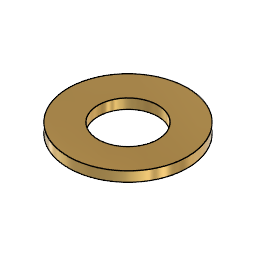
Parametric Shim (Autodesk Fusion 360 design; units mm, degrees)
part number: 3x6x.5mm Shim
Autodesk Fusion 360 part; units mm, degrees
sketch "Sketch1" plane through (0, 0, 0) normal (0, 0, 1) x (1, 0, 0)
  circle A0 centre (0, 0) radius 1.5
  circle A1 centre (0, 0) radius 3
  dimension "d1" = 3
  dimension "d5" = 6
  constraint coincident A0.centre A1.centre
  constraint concentric A0 A1
  measures "d1" diameter of A0
  measures "d5" diameter of A1
extrude "Extrude1" add sketch "Sketch1" along normal blind 0.5
equation "d1 = ID"
equation "ID = 3 mm"
equation "OD = 6 mm"
equation "Thickness = 0.5 mm"
equation "d5 = OD"
equation "d6 = Thickness"
